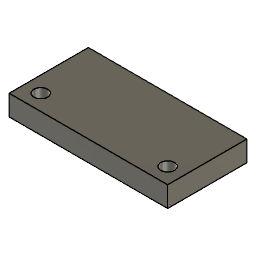
ToF_mount_v2 (Autodesk Fusion 360 design; units mm, degrees)
part number: 2026-02-15-15-34-03-763
Autodesk Fusion 360 part; units mm, degrees
sketch "Sketch1" plane through (0, 0, 0) normal (0, 0, 1) x (1, 0, 0)
  line L0 (-12.7, 7.3182) -> (12.7, 7.3182)
  line L1 (12.7, 7.3182) -> (12.7, -5.3818)
  line L2 (12.7, -5.3818) -> (-12.7, -5.3818)
  line L3 (-12.7, -5.3818) -> (-12.7, 7.3182)
  circle A0 centre (-10.16, -2.8418) radius 1.1
  circle A1 centre (10.16, -2.8418) radius 1.1
  dimension "d1" = 25.4
  dimension "d2" = 12.7
  dimension "d3" = 2.2
  dimension "d4" = 2.2
  dimension "d5" = 20.32
  dimension "d6" = 2.54
  dimension "d7" = 2.54
  dimension "d8" = 2.54
  constraint horizontal L0
  constraint vertical L1
  constraint horizontal L2
  constraint vertical L3
  measures "d1" distance of L0.start L0.end
  measures "d2" distance of L0.start L2.end
  measures "d3" diameter of A0
  measures "d4" diameter of A1
  measures "d5" distance of A0.centre A1.centre
  measures "d6" distance of L1 A1.centre
  measures "d7" distance of L3 A0.centre
  measures "d8" distance of L2 A0.centre
extrude "Extrude1" add sketch "Sketch1" along normal blind 6.35
extrude "Extrude2" cut 1 faces at (3.1179, 4.1809, 6.35) along direction (0, 0, -1) blind 3.048
